Autodesk Fusion 360 part; units mm, degrees
(part 3 of 3)
ref_plane "WorkPlane79" through (0, 0, -2.4) normal (0, 0, 1) x (1, 0, 0)
ref_plane "WorkPlane80" through (0, 0, -2.4) normal (0, 0, 1) x (1, 0, 0)
sketch "dp_disc" plane through (0, 0, 0) normal (0, 0, 1) x (1, 0, 0)
  line L0 (59.3, 26.1) -> (95.7, 26.1)
  line L1 (95.7, 26.1) -> (95.7, 37.9)
  line L2 (95.7, 37.9) -> (59.3, 37.9)
  line L3 (59.3, 37.9) -> (59.3, 26.1)
  line L4 (71.6, 13.8) -> (83.4, 13.8)
  line L5 (83.4, 13.8) -> (83.4, 50.2)
  line L6 (83.4, 50.2) -> (71.6, 50.2)
  line L7 (71.6, 50.2) -> (71.6, 13.8)
extrude "Extrude821" add sketch "dp_disc" along normal blind 2 separate body makes body 34
sketch "dp_skirt" plane through (0, 0, 0) normal (0, 0, 1) x (1, 0, 0)
  line L0 (59.8, 26.6) -> (95.2, 26.6)
  line L1 (95.2, 26.6) -> (95.2, 37.4)
  line L2 (95.2, 37.4) -> (59.8, 37.4)
  line L3 (59.8, 37.4) -> (59.8, 26.6)
  line L4 (72.1, 14.3) -> (82.9, 14.3)
  line L5 (82.9, 14.3) -> (82.9, 49.7)
  line L6 (82.9, 49.7) -> (72.1, 49.7)
  line L7 (72.1, 49.7) -> (72.1, 14.3)
extrude "Extrude822" add sketch "dp_skirt" against normal blind 2.4 bodies 34
sketch "dp_sk_820" plane through (0, 0, 0) normal (0, 0, 1) x (1, 0, 0)
  circle A0 centre (77.5, 45) radius 2.2
extrude "Extrude823" cut sketch "dp_sk_820" along normal blind 1.2 from surface at -2.4 bodies 34
sketch "dp_sk_794" plane through (0, 0, 0) normal (0, 0, 1) x (1, 0, 0)
  circle A0 centre (77.5, 19) radius 2.2
extrude "Extrude824" cut sketch "dp_sk_794" along normal blind 1.2 from surface at -2.4 bodies 34
sketch "dp_sk_677" plane through (0, 0, 0) normal (0, 0, 1) x (1, 0, 0)
  circle A0 centre (64.5, 32) radius 2.2
extrude "Extrude825" cut sketch "dp_sk_677" along normal blind 1.2 from surface at -2.4 bodies 34
sketch "dp_sk_937" plane through (0, 0, 0) normal (0, 0, 1) x (1, 0, 0)
  circle A0 centre (90.5, 32) radius 2.2
extrude "Extrude826" cut sketch "dp_sk_937" along normal blind 1.2 from surface at -2.4 bodies 34
sketch "dp_diag_0" plane through (0, 0, 0) normal (0, 0, 1) x (1, 0, 0)
  line L0 (71.6664, 25.8128) -> (83.6872, 37.8336)
  line L1 (83.6872, 37.8336) -> (83.3336, 38.1872)
  line L2 (83.3336, 38.1872) -> (71.3128, 26.1664)
  line L3 (71.3128, 26.1664) -> (71.6664, 25.8128)
extrude "Extrude827" cut sketch "dp_diag_0" along normal blind 0.6 from surface at 1.6 bodies 34
sketch "dp_diag_1" plane through (0, 0, 0) normal (0, 0, 1) x (1, 0, 0)
  line L0 (71.3128, 37.8336) -> (83.3336, 25.8128)
  line L1 (83.3336, 25.8128) -> (83.6872, 26.1664)
  line L2 (83.6872, 26.1664) -> (71.6664, 38.1872)
  line L3 (71.6664, 38.1872) -> (71.3128, 37.8336)
extrude "Extrude828" cut sketch "dp_diag_1" along normal blind 0.6 from surface at 1.6 bodies 34
sketch "dp_tri_U" plane through (0, 0, 0) normal (0, 0, 1) x (1, 0, 0)
  line L0 (77.5, 46.58) -> (74.98, 41.54)
  line L1 (74.98, 41.54) -> (80.02, 41.54)
  line L2 (80.02, 41.54) -> (77.5, 46.58)
extrude "Extrude829" cut sketch "dp_tri_U" along normal blind 0.6 from surface at 1.6 bodies 34
sketch "dp_tri_D" plane through (0, 0, 0) normal (0, 0, 1) x (1, 0, 0)
  line L0 (77.5, 17.42) -> (80.02, 22.46)
  line L1 (80.02, 22.46) -> (74.98, 22.46)
  line L2 (74.98, 22.46) -> (77.5, 17.42)
extrude "Extrude830" cut sketch "dp_tri_D" along normal blind 0.6 from surface at 1.6 bodies 34
sketch "dp_tri_L" plane through (0, 0, 0) normal (0, 0, 1) x (1, 0, 0)
  line L0 (62.92, 32) -> (67.96, 29.48)
  line L1 (67.96, 29.48) -> (67.96, 34.52)
  line L2 (67.96, 34.52) -> (62.92, 32)
extrude "Extrude831" cut sketch "dp_tri_L" along normal blind 0.6 from surface at 1.6 bodies 34
sketch "dp_tri_R" plane through (0, 0, 0) normal (0, 0, 1) x (1, 0, 0)
  line L0 (92.08, 32) -> (87.04, 34.52)
  line L1 (87.04, 34.52) -> (87.04, 29.48)
  line L2 (87.04, 29.48) -> (92.08, 32)
extrude "Extrude832" cut sketch "dp_tri_R" along normal blind 0.6 from surface at 1.6 bodies 34
sketch "np_d_Cap_pillA" plane through (0, 0, 0) normal (0, 0, 1) x (1, 0, 0)
  line L0 (30.7, 51.3) -> (45.3, 51.3)
  line L1 (45.3, 51.3) -> (45.3, 59.5)
  line L2 (45.3, 59.5) -> (30.7, 59.5)
  line L3 (30.7, 59.5) -> (30.7, 51.3)
extrude "Extrude833" add sketch "np_d_Cap_pillA" along normal blind 2 separate body makes body 35
ref_plane "WorkPlane81" through (0, 0, -2.4) normal (0, 0, 1) x (1, 0, 0)
sketch "np_st_Cap_pillA" plane through (0, 0, 0) normal (0, 0, 1) x (1, 0, 0)
  line L0 (30.75, 51.35) -> (45.25, 51.35)
  line L1 (45.25, 51.35) -> (45.25, 59.45)
  line L2 (45.25, 59.45) -> (30.75, 59.45)
  line L3 (30.75, 59.45) -> (30.75, 51.35)
sketch "np_sb_Cap_pillA" plane through (0, 0, -2.4) normal (0, 0, 1) x (1, 0, 0)
  line L0 (31.25, 51.85) -> (44.75, 51.85)
  line L1 (44.75, 51.85) -> (44.75, 58.95)
  line L2 (44.75, 58.95) -> (31.25, 58.95)
  line L3 (31.25, 58.95) -> (31.25, 51.85)
loft "Loft8" add profiles "np_st_Cap_pillA", "np_sb_Cap_pillA" section 1 section 2 bodies 35
sketch "np_sk_Cap_pillA" plane through (0, 0, 0) normal (0, 0, 1) x (1, 0, 0)
  circle A0 centre (38, 55.4) radius 2.5
extrude "Extrude834" cut sketch "np_sk_Cap_pillA" along normal blind 1 from surface at -2.4 bodies 35
fillet "Fillet58" radius 0.8 4 edges at (38, 59.5, 2) (45.3, 55.4, 2) (38, 51.3, 2) (30.7, 55.4, 2) on bodies 35
sketch "np_d_Cap_pillB" plane through (0, 0, 0) normal (0, 0, 1) x (1, 0, 0)
  line L0 (49.7, 51.3) -> (64.3, 51.3)
  line L1 (64.3, 51.3) -> (64.3, 59.5)
  line L2 (64.3, 59.5) -> (49.7, 59.5)
  line L3 (49.7, 59.5) -> (49.7, 51.3)
extrude "Extrude835" add sketch "np_d_Cap_pillB" along normal blind 2 separate body makes body 36
ref_plane "WorkPlane82" through (0, 0, -2.4) normal (0, 0, 1) x (1, 0, 0)
sketch "np_st_Cap_pillB" plane through (0, 0, 0) normal (0, 0, 1) x (1, 0, 0)
  line L0 (49.75, 51.35) -> (64.25, 51.35)
  line L1 (64.25, 51.35) -> (64.25, 59.45)
  line L2 (64.25, 59.45) -> (49.75, 59.45)
  line L3 (49.75, 59.45) -> (49.75, 51.35)
sketch "np_sb_Cap_pillB" plane through (0, 0, -2.4) normal (0, 0, 1) x (1, 0, 0)
  line L0 (50.25, 51.85) -> (63.75, 51.85)
  line L1 (63.75, 51.85) -> (63.75, 58.95)
  line L2 (63.75, 58.95) -> (50.25, 58.95)
  line L3 (50.25, 58.95) -> (50.25, 51.85)
loft "Loft9" add profiles "np_st_Cap_pillB", "np_sb_Cap_pillB" section 1 section 2 bodies 36
sketch "np_sk_Cap_pillB" plane through (0, 0, 0) normal (0, 0, 1) x (1, 0, 0)
  circle A0 centre (57, 55.4) radius 2.5
extrude "Extrude836" cut sketch "np_sk_Cap_pillB" along normal blind 1 from surface at -2.4 bodies 36
fillet "Fillet59" radius 0.8 4 edges at (57, 59.5, 2) (64.3, 55.4, 2) (57, 51.3, 2) (49.7, 55.4, 2) on bodies 36
extrude "Extrude850" add 4 faces at (90.9572, 32.7919, -1.2) (77.1333, 18.1463, -1.2) (65.0217, 33.0008, -1.2) (77.1333, 44.1463, -1.2) along direction (0, 0, -1) blind 1 on bodies 34 bodies 34
sketch "domeR_skirt" plane through (0, 0, 0) normal (0, 0, 1) x (1, 0, 0)
  circle A0 centre (19, 155) radius 11.15
extrude "Extrude851" add sketch "domeR_skirt" along normal blind 2.2 from surface at 5.8 separate body makes body 37
sketch "domeR_prof" plane through (0, 155, 0) normal (0, 1, 0) x (1, 0, 0)
  arc A0 (19, -12) -> (29, -8) centre (19, 2.5) ccw
  line L0 (29, -8) -> (19, -8)
  line L1 (19, -8) -> (19, -12)
revolve "Revolve5" add sketch "domeR_prof" angle 360 about axis through (19, 155, 8) along (0, 0, 1) bodies 37
shell "Shell14" thickness 1.5 removed faces 1 at (24.0027, 153.3874, 5.8) on bodies 37
extrude "Extrude837" [suppressed]
extrude "Extrude838" [suppressed]
extrude "Extrude839" [suppressed]
extrude "Extrude840" [suppressed]
extrude "Extrude841" [suppressed]
extrude "Extrude842" [suppressed]
extrude "Extrude843" [suppressed]
sketch "Sketch725" plane through (0, 14.3, 0) normal (0, -1, 0) x (1, 0, 0)
  line L0 (72.6, 0) -> (72.6, -2.4)
  line L1 (72.6, -2.4) -> (82.9, -2.4)
  line L2 (82.9, -2.4) -> (82.9, 0)
  line L3 (82.9, 0) -> (72.6, 0)
extrude "Extrude844" [suppressed]
extrude "Extrude845" [suppressed]
extrude "Extrude846" [suppressed]
extrude "Extrude847" [suppressed]
extrude "Extrude848" [suppressed]
extrude "Extrude849" [suppressed]
equation "ShellThickness = 2.5 mm" comment "outer wall"
equation "RibThickness = 2.0 mm" comment "internal ribs"
equation "Tolerance = 0.25 mm" comment "general fit clearance"
equation "BodyWidth = 112 mm" comment "left half width"
equation "BodyHeight = 170 mm" comment "overall height"
equation "BodyDepth = 27 mm" comment "left half depth"
equation "RightWidth = 104 mm" comment "right half width"
equation "RightDepth = 15 mm" comment "right half depth"
equation "TopCurveDrop = 34 mm" comment "curved top profile drop"
equation "CornerFillet = 7 mm" comment "body corner fillet"
equation "EdgeFillet = 3 mm" comment "shell edge fillet"
equation "HingeDiameter = 16 mm" comment "hinge barrel OD"
equation "HingePinDia = 3 mm" comment "metal hinge pin"
equation "HingeGap = 0.4 mm" comment "hinge knuckle gap"
equation "DisplayW = 47.3 mm" comment "waveshare 2.8 active W"
equation "DisplayH = 79 mm" comment "waveshare 2.8 active H"
equation "DisplayOffset = 2.0 mm" comment "display below bezel face"
equation "BezelWidth = 9 mm" comment "white bezel border"
equation "CameraDia = 22 mm" comment "camera lens dome dia"
equation "CameraDepth = 9 mm" comment "camera module recess"
equation "LedDia = 4.5 mm" comment "status LED window"
equation "ButtonTravel = 0.9 mm" comment "plunger travel"
equation "ButtonClear = 0.35 mm" comment "plunger to guide clearance"
equation "BatteryDiameter = 21.5 mm" comment "INR21700 dia + tol"
equation "BatteryLength = 70.5 mm" comment "INR21700 length + tol"
equation "SpeakerDia = 40 mm" comment "speaker OD"
equation "SpeakerDepth = 6 mm" comment "speaker chamber depth"
equation "PCBOffset = 4 mm" comment "PCB standoff height"
equation "InsertDiameter = 4.2 mm" comment "M3 brass insert hole"
equation "InsertDepth = 5.5 mm" comment "insert depth"
equation "BossDiameter = 7 mm" comment "boss OD"
equation "ScrewClearance = 3.4 mm" comment "M3 clearance hole"
equation "WireChannelWidth = 5 mm" comment "cable channel"
equation "VentSlotW = 1.6 mm" comment "vent slot width"
equation "LensBossDia = 34 mm" comment "camera dome boss outer dia"
equation "LensBossH = 9 mm" comment "camera dome height above shell"
equation "ShoulderRise = 30 mm" comment "height of raised lens shoulder above body top"
equation "CurveStartFrac = 0.46" comment "fraction of right width where S-curve starts"
equation "lcd_thk = 8 mm" comment "LCD module thickness glass front to PCB back - MEASURE AND EDIT"
equation "d379 = -lcd_thk - 2 mm"
equation "d381 = -lcd_thk"
equation "d383 = -lcd_thk + 4.5 mm"
equation "d386 = -6.4 mm - lcd_thk"
equation "d392 = -5.6 mm - lcd_thk"
equation "d398 = -lcd_thk - 2 mm"
equation "d400 = -lcd_thk + 2.5 mm"
equation "cam_pair = 4.2 mm" comment "OV5693 right pair hole spacing - VERIFY vs PCB"
equation "cam_lens = 5.45 mm" comment "OV5693 VCM lens height above PCB"
equation "d473 = cam_lens - 3 mm"
equation "d487 = cam_lens - 3 mm"
equation "btn_switch_h = 13 mm" comment "6x6x8 switch: body 8 + plunger 5 = tip-to-board"
equation "btn_board_t = 1.6 mm" comment "perfboard thickness"
equation "btn_gap = 2 mm" comment "plunger tip clearance behind front wall"
equation "btn_wall = 6.4 mm" comment "front face to inner wall (=wall+field)"
equation "btn_standoff_h = 14 mm" comment "standoff height (board seat below inner wall) - TUNE THIS"
equation "d752 = -btn_standoff_h"
equation "d754 = -btn_standoff_h"
equation "d756 = -btn_standoff_h"
equation "d758 = -btn_standoff_h"
equation "d760 = -btn_standoff_h"
equation "d762 = -btn_standoff_h"
equation "d764 = -btn_standoff_h"
equation "d767 = -btn_standoff_h"
equation "d770 = -btn_standoff_h"
equation "d773 = -btn_standoff_h"
equation "d776 = -btn_standoff_h"
equation "d779 = -btn_standoff_h"
named bodies: "LeftTub", "BackPlate", "RightLid", "LidFacePlate", "LCDCrossPlate", "Dummy_Screen_R", "DummyKey_Top_157", "DummyKey_Top_172", "DummyKey_Top_142", "DummyKey_Top_187", "DummyKey_Top_202", "DummyKey_Bot_157", "DummyKey_Bot_187", "DummyKey_Bot_142", "DummyKey_Bot_172", "DummyKey_Bot_202", "DummyBtn_Small_142", "DummyBtn_Small_155", "DummyBtn_Mute", "DummyBtn_Wide_139", "DummyBtn_Wide_190", "DummyPill_186", "DummyPill_202", "ArduinoMount", "ScreenBezel", "Dome_Lens", "Dome_Ring", "Cap_Back", "Cap_btn9", "Cap_Select", "Cap_DPad", "Cap_pillA", "Cap_pillB"
